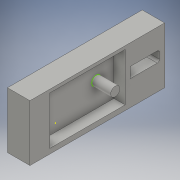
# Autodesk Inventor part: 7.2 part 1
Saved by Autodesk Inventor 2016 (Build 200138000, 138)
## iProperties
Created: 2017-03-14
Part Number: 7.2 part 1
Material: Generic
Document SubType Name: Modeling
Designer: 196918
Density: 1 g/cm^3
Appearance: Default
Author: 196918
Autodesk Inventor part; units mm, degrees
ref_plane "YZ Plane" through (0, 0, 0) normal (1, 0, 0) x (0, 1, 0)
ref_plane "XZ Plane" through (0, 0, 0) normal (0, 1, 0) x (-1, 0, 0)
ref_plane "XY Plane" through (0, 0, 0) normal (0, 0, 1) x (1, 0, 0)
sketch "Sketch1" plane through (0, 0, 0) normal (1, 0, 0) x (0, 1, 0)
  line L0 (-7.2949, 20.7328) -> (24.4551, 20.7328)
  line L1 (24.4551, 20.7328) -> (24.4551, -55.4672)
  line L2 (24.4551, -55.4672) -> (-7.2949, -55.4672)
  line L3 (-7.2949, -55.4672) -> (-7.2949, 20.7328)
  point P0 (0, 0)
  dimension "d0" = 31.75
  dimension "d1" = 76.2
  constraints: 8 end point, 2 parallel, 1 horizontal, 1 perpendicular
  measures "d0" distance of L1.end L2.end
  measures "d1" distance of L0.end L1.end
extrude "Extrusion1" add sketch "Sketch1" along normal blind 12.7
sketch "Sketch2" plane through (12.7, 0, 0) normal (1, 0, 0) x (0, 0, -1)
  line L0 (-9.5129, 22.6408) -> (33.105, 22.6408)
  line L1 (33.105, 22.6408) -> (33.105, -4.5028)
  line L2 (33.105, -4.5028) -> (-9.5129, -4.5028)
  line L3 (-9.5129, -4.5028) -> (-9.5129, 22.6408)
  line L4 (35.8954, 12.8742) -> (52.5113, 12.8742)
  line L5 (52.5113, 12.8742) -> (52.5113, 6.9127)
  line L6 (52.5113, 6.9127) -> (35.8954, 6.9127)
  line L7 (35.8954, 6.9127) -> (35.8954, 12.8742)
  point P0 (0, 0)
  constraints: 16 end point, 4 parallel, 2 horizontal, 2 perpendicular
extrude "Extrusion2" cut sketch "Sketch2" against normal blind 6.35
fillet "Fillet1" radius 1.27 2 edges at (9.525, 12.8742, -52.5113) (9.525, 6.9127, -52.5113)
sketch "Sketch3" plane through (6.35, 0, 0) normal (1, 0, 0) x (0, 0, -1)
  circle A0 centre (23.0847, 9.3227) radius 2.6025
  circle A1 centre (-4.0588, 9.3227) radius 0.761
  point P0 (0, 0)
  constraints: 2 centre point
extrude "Extrusion3" cut sketch "Sketch3" against normal blind 1.27 contours A1
extrude "Extrusion4" add sketch "Sketch3" along normal blind 10.795 contours A0
body "Solid1"
